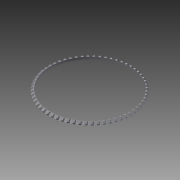
# Autodesk Inventor part: InnerPivotalRing
Saved by Autodesk Inventor 2015 (Build 190159000, 159)
## iProperties
Created: 2015-06-16
Part Number: InnerPivotalRing
Material: Generic
Document SubType Name: Modeling
Designer: david_000
Density: 1 g/cm^3
Appearance: Default
Author: david_000
Autodesk Inventor part; units mm, degrees
ref_plane "YZ Plane" through (0, 0, 0) normal (1, 0, 0) x (0, 1, 0)
ref_plane "XZ Plane" through (0, 0, 0) normal (0, 1, 0) x (-1, 0, 0)
ref_plane "XY Plane" through (0, 0, 0) normal (0, 0, 1) x (1, 0, 0)
sketch "Sketch2" plane through (0, 0, 0) normal (0, 1, 0) x (-1, 0, 0)
  line L0 (-48.0642, 4.5226) -> (-47.7617, 7.0319)
  line L1 (-47.7617, 7.0319) -> (-47.3282, 9.522)
  line L2 (-47.3282, 9.522) -> (-46.765, 11.9859)
  line L3 (-46.765, 11.9859) -> (-46.0736, 14.4169)
  line L4 (-46.0736, 14.4169) -> (-45.2559, 16.8085)
  line L5 (-45.2559, 16.8085) -> (-44.3142, 19.154)
  line L6 (-44.3142, 19.154) -> (-43.2511, 21.4469)
  line L7 (-43.2511, 21.4469) -> (-42.0693, 23.6811)
  line L8 (-42.0693, 23.6811) -> (-40.7723, 25.8504)
  line L9 (-40.7723, 25.8504) -> (-39.3635, 27.9488)
  line L10 (-39.3635, 27.9488) -> (-37.8468, 29.9707)
  line L11 (-37.8468, 29.9707) -> (-36.2264, 31.9103)
  line L12 (-36.2264, 31.9103) -> (-34.5067, 33.7626)
  line L13 (-34.5067, 33.7626) -> (-32.6924, 35.5222)
  line L14 (-32.6924, 35.5222) -> (-30.7885, 37.1845)
  line L15 (-30.7885, 37.1845) -> (-28.8003, 38.7449)
  line L16 (-28.8003, 38.7449) -> (-26.733, 40.1991)
  line L17 (-26.733, 40.1991) -> (-24.5925, 41.5431)
  line L18 (-24.5925, 41.5431) -> (-22.3846, 42.7733)
  line L19 (-22.3846, 42.7733) -> (-20.1154, 43.8862)
  line L20 (-20.1154, 43.8862) -> (-17.791, 44.8788)
  line L21 (-17.791, 44.8788) -> (-15.4178, 45.7484)
  line L22 (-15.4178, 45.7484) -> (-13.0024, 46.4926)
  line L23 (-13.0024, 46.4926) -> (-10.5514, 47.1094)
  line L24 (-10.5514, 47.1094) -> (-8.0714, 47.597)
  line L25 (-8.0714, 47.597) -> (-5.5693, 47.9542)
  line L26 (-5.5693, 47.9542) -> (-3.0519, 48.18)
  line L27 (-3.0519, 48.18) -> (-0.5262, 48.2737)
  line L28 (-0.5262, 48.2737) -> (2.001, 48.2351)
  line L29 (2.001, 48.2351) -> (4.5226, 48.0642)
  line L30 (4.5226, 48.0642) -> (7.0319, 47.7617)
  line L31 (7.0319, 47.7617) -> (9.522, 47.3282)
  line L32 (9.522, 47.3282) -> (11.9859, 46.765)
  line L33 (11.9859, 46.765) -> (14.4169, 46.0736)
  line L34 (14.4169, 46.0736) -> (16.8085, 45.2559)
  line L35 (16.8085, 45.2559) -> (19.154, 44.3142)
  line L36 (19.154, 44.3142) -> (21.4469, 43.2511)
  line L37 (21.4469, 43.2511) -> (23.6811, 42.0693)
  line L38 (23.6811, 42.0693) -> (25.8504, 40.7723)
  line L39 (25.8504, 40.7723) -> (27.9488, 39.3635)
  line L40 (27.9488, 39.3635) -> (29.9707, 37.8468)
  line L41 (29.9707, 37.8468) -> (31.9103, 36.2264)
  line L42 (31.9103, 36.2264) -> (33.7626, 34.5067)
  line L43 (33.7626, 34.5067) -> (35.5222, 32.6924)
  line L44 (35.5222, 32.6924) -> (37.1845, 30.7885)
  line L45 (37.1845, 30.7885) -> (38.7449, 28.8003)
  line L46 (38.7449, 28.8003) -> (40.1991, 26.733)
  line L47 (40.1991, 26.733) -> (41.5431, 24.5925)
  line L48 (41.5431, 24.5925) -> (42.7733, 22.3846)
  line L49 (42.7733, 22.3846) -> (43.8862, 20.1154)
  line L50 (43.8862, 20.1154) -> (44.8788, 17.791)
  line L51 (44.8788, 17.791) -> (45.7484, 15.4178)
  line L52 (45.7484, 15.4178) -> (46.4926, 13.0024)
  line L53 (46.4926, 13.0024) -> (47.1094, 10.5514)
  line L54 (47.1094, 10.5514) -> (47.597, 8.0714)
  line L55 (47.597, 8.0714) -> (47.9542, 5.5693)
  line L56 (47.9542, 5.5693) -> (48.18, 3.0519)
  line L57 (48.18, 3.0519) -> (48.2737, 0.5262)
  line L58 (48.2737, 0.5262) -> (48.2351, -2.001)
  line L59 (48.2351, -2.001) -> (48.0642, -4.5226)
  line L60 (48.0642, -4.5226) -> (47.7617, -7.0319)
  line L61 (47.7617, -7.0319) -> (47.3282, -9.522)
  line L62 (47.3282, -9.522) -> (46.765, -11.9859)
  line L63 (46.765, -11.9859) -> (46.0736, -14.4169)
  line L64 (46.0736, -14.4169) -> (45.2559, -16.8085)
  line L65 (45.2559, -16.8085) -> (44.3142, -19.154)
  line L66 (44.3142, -19.154) -> (43.2511, -21.4469)
  line L67 (43.2511, -21.4469) -> (42.0693, -23.6811)
  line L68 (42.0693, -23.6811) -> (40.7723, -25.8504)
  line L69 (40.7723, -25.8504) -> (39.3635, -27.9488)
  line L70 (39.3635, -27.9488) -> (37.8468, -29.9707)
  line L71 (37.8468, -29.9707) -> (36.2264, -31.9103)
  line L72 (36.2264, -31.9103) -> (34.5067, -33.7626)
  line L73 (34.5067, -33.7626) -> (32.6924, -35.5222)
  line L74 (32.6924, -35.5222) -> (30.7885, -37.1845)
  line L75 (30.7885, -37.1845) -> (28.8003, -38.7449)
  line L76 (28.8003, -38.7449) -> (26.733, -40.1991)
  line L77 (26.733, -40.1991) -> (24.5925, -41.5431)
  line L78 (24.5925, -41.5431) -> (22.3846, -42.7733)
  line L79 (22.3846, -42.7733) -> (20.1154, -43.8862)
  line L80 (20.1154, -43.8862) -> (17.791, -44.8788)
  line L81 (17.791, -44.8788) -> (15.4178, -45.7484)
  line L82 (15.4178, -45.7484) -> (13.0024, -46.4926)
  line L83 (13.0024, -46.4926) -> (10.5514, -47.1094)
  line L84 (10.5514, -47.1094) -> (8.0714, -47.597)
  line L85 (8.0714, -47.597) -> (5.5693, -47.9542)
  line L86 (5.5693, -47.9542) -> (3.0519, -48.18)
  line L87 (3.0519, -48.18) -> (0.5262, -48.2737)
  line L88 (0.5262, -48.2737) -> (-2.001, -48.2351)
  line L89 (-2.001, -48.2351) -> (-4.5226, -48.0642)
  line L90 (-4.5226, -48.0642) -> (-7.0319, -47.7617)
  line L91 (-7.0319, -47.7617) -> (-9.522, -47.3282)
  line L92 (-9.522, -47.3282) -> (-11.9859, -46.765)
  line L93 (-11.9859, -46.765) -> (-14.4169, -46.0736)
  line L94 (-14.4169, -46.0736) -> (-16.8085, -45.2559)
  line L95 (-16.8085, -45.2559) -> (-19.154, -44.3142)
  line L96 (-19.154, -44.3142) -> (-21.4469, -43.2511)
  line L97 (-21.4469, -43.2511) -> (-23.6811, -42.0693)
  line L98 (-23.6811, -42.0693) -> (-25.8504, -40.7723)
  line L99 (-25.8504, -40.7723) -> (-27.9488, -39.3635)
  line L100 (-27.9488, -39.3635) -> (-29.9707, -37.8468)
  line L101 (-29.9707, -37.8468) -> (-31.9103, -36.2264)
  line L102 (-31.9103, -36.2264) -> (-33.7626, -34.5067)
  line L103 (-33.7626, -34.5067) -> (-35.5222, -32.6924)
  line L104 (-35.5222, -32.6924) -> (-37.1845, -30.7885)
  line L105 (-37.1845, -30.7885) -> (-38.7449, -28.8003)
  line L106 (-38.7449, -28.8003) -> (-40.1991, -26.733)
  line L107 (-40.1991, -26.733) -> (-41.5431, -24.5925)
  line L108 (-41.5431, -24.5925) -> (-42.7733, -22.3846)
  line L109 (-42.7733, -22.3846) -> (-43.8862, -20.1154)
  line L110 (-43.8862, -20.1154) -> (-44.8788, -17.791)
  line L111 (-44.8788, -17.791) -> (-45.7484, -15.4178)
  line L112 (-45.7484, -15.4178) -> (-46.4926, -13.0024)
  line L113 (-46.4926, -13.0024) -> (-47.1094, -10.5514)
  line L114 (-47.1094, -10.5514) -> (-47.597, -8.0714)
  line L115 (-47.597, -8.0714) -> (-47.9542, -5.5693)
  line L116 (-47.9542, -5.5693) -> (-48.18, -3.0519)
  line L117 (-48.18, -3.0519) -> (-48.2737, -0.5262)
  line L118 (-48.2737, -0.5262) -> (-48.2351, 2.001)
  line L119 (-48.2351, 2.001) -> (-48.0642, 4.5226)
  point P0 (0, 0)
  point P1 (0, 0)
  dimension "d11" = 96.52
  constraints: 240 end point, 241 other
  measures "d11" distance between parallel lines of L57 L117
extrude "Extrusion2" add sketch "Sketch2" along normal blind 76.2 draft -45
sketch "Sketch3" plane through (0, 0, 0) normal (0, -1, 0) x (1, 0, 0)
  circle A0 centre (0, 0) radius 45.72
  dimension "d14" = 91.44
  constraints: 1 centre point, 1 coincident
  measures "d14" diameter of A0
extrude "Extrusion3" cut sketch "Sketch3" against normal blind 76.2
sketch "Sketch4" plane through (-7.0319, 0, 47.7617) normal (-0.0846491, 0.7071068, 0.7020217) x (0.9928087, 0, 0.1197118)
  line L0 (0, 0) -> (2.4605, 0)
  line L1 (2.4605, 0) -> (2.4605, 3.6143)
  line L2 (2.4605, 3.6143) -> (0, 3.6143)
  line L3 (0, 3.6143) -> (0, 0)
  point P0 (1.2637, 34.125)
  constraints: 8 end point, 2 parallel, 1 horizontal, 1 perpendicular
extrude "Extrusion4" add sketch "Sketch4" along normal blind 1.27 draft -30
pattern_circular "Circular Pattern1" count 60 over 360 about axis through (0, 0, 0) along (0, 1, 0) of "Extrusion4"
body "Solid2"
